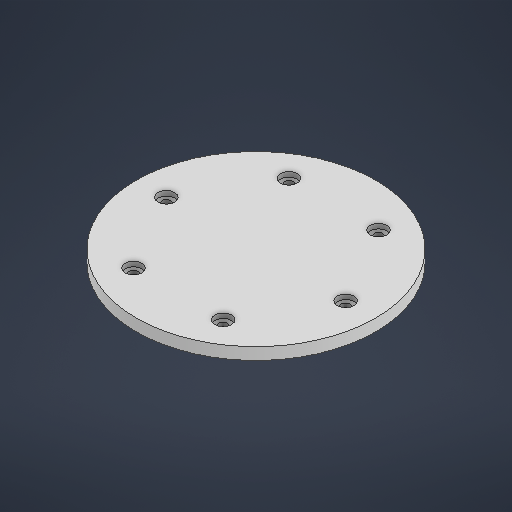
# Autodesk Inventor part: Pieza8
Saved by Autodesk Inventor 2026.1 (Build 301233000, 233)
## iProperties
Created: 2025-09-20
Part Number: Pieza8
Material: Genérico
Document SubType Name: Modeling
Designer: Usuario
Density: 1 g/cm^3
Appearance: Valor por defecto
Author: Usuario
Autodesk Inventor part; units mm, degrees
ref_plane "YZ Plane" through (0, 0, 0) normal (1, 0, 0) x (0, 1, 0)
ref_plane "XZ Plane" through (0, 0, 0) normal (0, 1, 0) x (-1, 0, 0)
ref_plane "XY Plane" through (0, 0, 0) normal (0, 0, 1) x (1, 0, 0)
sketch "Boceto1" plane through (0, 0, 0) normal (0, 1, 0) x (-1, 0, 0)
  circle A0 centre (0, 0) radius 50
  dimension "d0" = 100
  constraints: 1 centre point, 1 coincident
  measures "d0" diameter of A0
extrude "Extrusión1" add sketch "Boceto1" along normal blind 5
sketch "Boceto2" plane through (0, 5, 0) normal (0, 1, 0) x (1, 0, 0)
  circle A0 centre (0, 0) radius 37.5 construction
  line L0 (-37.5, 0) -> (-18.75, 32.476) construction
  line L1 (-18.75, 32.476) -> (18.75, 32.476) construction
  line L2 (18.75, 32.476) -> (37.5, 0) construction
  line L3 (37.5, 0) -> (18.75, -32.476) construction
  line L4 (18.75, -32.476) -> (-18.75, -32.476) construction
  line L5 (-18.75, -32.476) -> (-37.5, 0) construction
  circle A1 centre (-18.75, -32.476) radius 3.5
  circle A2 centre (-37.5, 0) radius 3.5
  circle A3 centre (-18.75, 32.476) radius 3.5
  circle A4 centre (18.75, 32.476) radius 3.5
  circle A5 centre (37.5, 0) radius 3.5
  circle A6 centre (18.75, -32.476) radius 3.5
  dimension "d3" = 75
  dimension "d4" = 7
  dimension "d5" = 7
  dimension "d6" = 7
  dimension "d7" = 7
  dimension "d8" = 7
  dimension "d9" = 7
  constraints: 12 end point, 8 coincident, 6 centre point, 1 horizontal alignment, 15 other
  measures "d4" diameter of A1
  measures "d5" diameter of A2
  measures "d6" diameter of A3
  measures "d7" diameter of A4
  measures "d8" diameter of A5
  measures "d9" diameter of A6
extrude "Extrusión2" cut sketch "Boceto2" against normal blind 2
sketch "Boceto3" plane through (0, 5, 0) normal (0, 1, 0) x (1, 0, 0)
  circle A0 centre (0, 0) radius 37.5 construction
  circle A1 centre (37.5, 0) radius 3.5 projected
  line L0 (37.5, 0) -> (18.75, -32.476) construction
  line L1 (18.75, -32.476) -> (-18.75, -32.476) construction
  line L2 (-18.75, -32.476) -> (-37.5, 0) construction
  line L3 (-37.5, 0) -> (-18.75, 32.476) construction
  line L4 (-18.75, 32.476) -> (18.75, 32.476) construction
  line L5 (18.75, 32.476) -> (37.5, 0) construction
  circle A2 centre (-37.5, 0) radius 1.75
  circle A3 centre (-18.75, -32.476) radius 1.75
  circle A4 centre (18.75, -32.476) radius 1.75
  circle A5 centre (37.5, 0) radius 1.75
  circle A6 centre (18.75, 32.476) radius 1.75
  circle A7 centre (-18.75, 32.476) radius 1.75
  dimension "d12" = 75
  dimension "d13" = 3.5
  dimension "d14" = 3.5
  dimension "d15" = 3.5
  dimension "d16" = 3.5
  dimension "d17" = 3.5
  dimension "d18" = 3.5
  constraints: 12 end point, 7 centre point, 7 coincident, 1 point on line, 13 other
  measures "d12" diameter of A0
  measures "d13" diameter of A2
  measures "d14" diameter of A3
  measures "d15" diameter of A4
  measures "d16" diameter of A5
  measures "d17" diameter of A6
  measures "d18" diameter of A7
extrude "Extrusión3" cut sketch "Boceto3" along normal mid plane 10 contours A2 | A3 | A4 | A5 | A6 | A7
